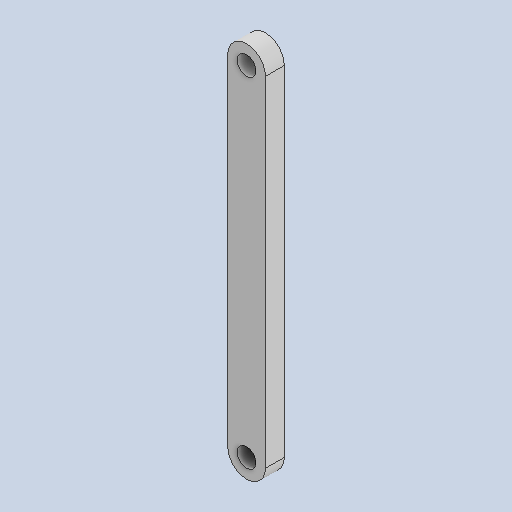
# Autodesk Inventor part: legparts_03(six)
Saved by Autodesk Inventor 2024.3 (Build 283343000, 343)
## iProperties
Created: 2024-10-20
Part Number: legparts_03(six)
Material: 一般
Document SubType Name: Modeling
Designer: 佐藤智貴
Density: 1 g/cm^3
Appearance: 既定
Mass: 144.641 g
Surface Area: 171.708 cm^2
Volume: 53.5708 cm^3
Author: 佐藤智貴
Autodesk Inventor part; units mm, degrees
ref_plane "YZ Plane" through (0, 0, 0) normal (1, 0, 0) x (0, 1, 0)
ref_plane "XZ Plane" through (0, 0, 0) normal (0, 1, 0) x (-1, 0, 0)
ref_plane "XY Plane" through (0, 0, 0) normal (0, 0, 1) x (1, 0, 0)
sketch "スケッチ1" plane through (0, 0, 0) normal (0, 0, 1) x (1, 0, 0)
  circle A0 centre (0, 0) radius 5
  circle A1 centre (0, 0) radius 10
  line L0 (-5, 0) -> (5, 0)
  line L1 (5, 0) -> (5, -190)
  line L2 (5, -190) -> (-5, -190)
  line L3 (-5, -190) -> (-5, 0)
  line L4 (-10, 0) -> (-10, -190)
  line L5 (-10, -190) -> (5, -190)
  line L6 (10, 0) -> (10, -190)
  line L7 (10, -190) -> (5, -190)
  circle A2 centre (0, -180) radius 5
  circle A3 centre (0, -180) radius 10
  point P0 (5, -8.6603)
  point P1 (-5, -8.6603)
  point P2 (-5, -171.3397)
  point P3 (5, -171.3397)
  point P4 (-10, -180)
  point P5 (10, -180)
  dimension "d0" = 10
  dimension "d1" = 20
  dimension "d3" = 10
  dimension "d15" = 20
  dimension "d16" = 10
  dimension "d17" = 20
  dimension "d18" = 10
  dimension "d19" = 10
  dimension "d22" = 180
  constraints: 16 end point, 4 parallel, 3 centre point, 3 perpendicular, 2 point on circle, 1 coincident, 1 horizontal, 1 horizontal alignment, 1 point on line, 1 tangent, 2 other
  measures "d1" diameter of A1
  measures "d3" distance of L0.start L0.end
  measures "d15" distance between parallel lines of L6 L4
  measures "d16" diameter of A2
  measures "d17" diameter of A3
  measures "d18" distance from line of L5 A2.centre
  measures "d19" distance from line of L4 A2.centre
  measures "d22" distance of A2.centre A1.centre
extrude "押し出し1" add sketch "スケッチ1" along normal blind 10 contours L1 A1 L3 A0 | A0 L3 A1 L1 | L1 A3 L3 A1 | A1 L6 A3 L1 | L3 A3 L4 A1 | A3 L1 | L1 A2 L3 A3 | L3 A3 | L1 A3 L3 A2
